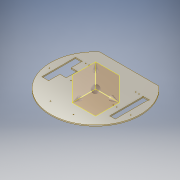
# Autodesk Inventor part: BottomPlate
Saved by Autodesk Inventor 2019 (Build 230136000, 136)
## iProperties
Created: 2020-02-28
Part Number: BottomPlate
Material: Generic
Document SubType Name: Modeling
Designer: james
Mass: 617.778 g
Surface Area: 2655.15 cm^2
Volume: 617.778 cm^3
Density: 1 g/cm^3
Appearance: Titanium
Author: james
Autodesk Inventor part; units mm, degrees
ref_plane "YZ Plane" through (0, 0, 0) normal (1, 0, 0) x (0, 1, 0)
ref_plane "XZ Plane" through (0, 0, 0) normal (0, 1, 0) x (-1, 0, 0)
ref_plane "XY Plane" through (0, 0, 0) normal (0, 0, 1) x (1, 0, 0)
sketch "Sketch1" plane through (0, 0, 0) normal (0, 1, 0) x (-1, 0, 0)
  circle A0 centre (0, 0) radius 203.2
  dimension "d0" = 406.4
  constraints: 1 centre point, 1 coincident
  measures "d0" diameter of A0
extrude "Extrusion1" add sketch "Sketch1" along normal blind 4.7625
sketch "Sketch2" plane through (0, 4.7625, 0) normal (0, 1, 0) x (1, 0, 0)
  line L0 (-165.1, -76.2) -> (-139.7, -76.2)
  line L1 (-139.7, -76.2) -> (-139.7, 76.2)
  line L2 (-139.7, 76.2) -> (-165.1, 76.2)
  line L3 (-165.1, 76.2) -> (-165.1, -76.2)
  line L4 (139.7, 76.2) -> (165.1, 76.2)
  line L5 (165.1, 76.2) -> (165.1, -76.2)
  line L6 (165.1, -76.2) -> (139.7, -76.2)
  line L7 (139.7, -76.2) -> (139.7, 76.2)
  point P0 (0, 0)
  dimension "d3" = 25.4
  dimension "d4" = 25.4
  dimension "d5" = 0
  dimension "d6" = 0
  dimension "d7" = 152.4
  dimension "d8" = 76.2
  dimension "d9" = 139.7
  dimension "d10" = 139.7
  constraints: 16 end point, 4 parallel, 2 horizontal, 2 perpendicular
  measures "d3" distance of L5.end L6.end
  measures "d4" distance of L0.start L0.end
  measures "d5" distance between parallel lines of L6 L0
  measures "d6" distance between parallel lines of L4 L2
  measures "d7" distance of L4.end L5.end
  measures "d8" distance from line of point (0, 0) L6
  measures "d9" distance from line of L1 point (0, 0)
  measures "d10" distance from line of L7 point (0, 0)
extrude "Extrusion2" cut sketch "Sketch2" against normal blind 28.575
sketch "Sketch3" plane through (0, 4.7625, 0) normal (0, 1, 0) x (1, 0, 0)
  line L0 (-139.7, 76.2) -> (-139.7, -76.2) projected
  line L1 (-139.7, -76.2) -> (-165.1, -76.2) projected
  line L2 (-139.7, 76.2) -> (-165.1, 76.2) projected
  point P0 (0, 0)
  point P1 (-120.65, 76.2)
  dimension "d30" = 0
  dimension "d90" = 19.05
  measures "d30" distance from line of point (-120.65, 76.2) L2
  measures "d90" distance from line of L0 point (-120.65, 76.2)
hole "Hole1" at (-120.65, 4.7625, -76.2) direction (0, -1, 0) diameter 3.81 depth 25.4 tip angle 118
sketch "Sketch4" plane through (0, 0, 0) normal (0, -1, 0) x (1, 0, 0)
  line L0 (-136.525, 76.2) -> (-167.64, 76.2)
  line L1 (-167.64, 76.2) -> (-167.64, -76.2)
  line L2 (-167.64, -76.2) -> (-136.525, -76.2)
  line L3 (-136.525, -76.2) -> (-136.525, 76.2)
  line L4 (-139.7, -76.2) -> (-165.1, -76.2) projected
  line L5 (-165.1, 76.2) -> (-139.7, 76.2) projected
  line L6 (-165.1, -76.2) -> (-165.1, 76.2) projected
  line L7 (-139.7, 76.2) -> (-139.7, -76.2) projected
  point P0 (0, 0)
  dimension "d24" = 0
  dimension "d25" = 0
  dimension "d26" = 2.54
  dimension "d27" = 3.175
  constraints: 8 end point, 2 parallel, 1 horizontal, 1 perpendicular
  measures "d24" distance between parallel lines of L2 L4
  measures "d25" distance between parallel lines of L5 L0
  measures "d26" distance between parallel lines of L6 L1
  measures "d27" distance between parallel lines of L7 L3
extrude "Extrusion3" cut sketch "Sketch4" against normal blind 11.1125 contours L3 L2 L7 L0 | L6 L2 L1 L0
sketch "Sketch5" plane through (0, 0, 0) normal (0, -1, 0) x (1, 0, 0)
  circle A0 centre (-120.65, 25.4) radius 1.905 projected
  circle A1 centre (-120.65, -76.2) radius 1.905 projected
  point P0 (0, 0)
  point P1 (-86.36, 25.4)
  point P2 (-105.41, -76.2)
  point P3 (-184.15, 25.4)
  dimension "d33" = 0
  dimension "d34" = 15.24
  dimension "d88" = 101.6
  dimension "d91" = 97.79
  measures "d33" vertical distance of A1.centre point (-105.41, -76.2)
  measures "d34" distance of A1.centre point (-105.41, -76.2)
  measures "d88" vertical distance of point (-184.15, 25.4) A1.centre
  measures "d91" distance of point (-184.15, 25.4) point (-86.36, 25.4)
hole "Hole2" at (-86.36, 0, 25.4) at (-105.41, 0, -76.2) at (-184.15, 0, 25.4) direction (0, 1, 0) diameter 3.81 depth 25.4 tip angle 118
sketch "Sketch6" plane through (0, 0, 0) normal (0, -1, 0) x (1, 0, 0)
  point P0 (0, 0)
  point P1 (52.197, 152.4)
  point P2 (-52.197, 152.4)
  dimension "d48" = 0
  dimension "d49" = 104.394
  dimension "d50" = 52.197
  dimension "d51" = 152.4
  measures "d48" vertical distance of point (-52.197, 152.4) point (52.197, 152.4)
  measures "d49" distance of point (-52.197, 152.4) point (52.197, 152.4)
  measures "d50" horizontal distance of point (0, 0) point (52.197, 152.4)
  measures "d51" vertical distance of point (0, 0) point (-52.197, 152.4)
hole "Hole3" at (52.197, 0, 152.4) at (-52.197, 0, 152.4) direction (0, 1, 0) diameter 3.81 depth 25.4 tip angle 118
sketch "Sketch7" plane through (0, 0, 0) normal (0, -1, 0) x (1, 0, 0)
  circle A0 centre (-86.36, 25.4) radius 1.905 projected
  circle A1 centre (-120.65, 25.4) radius 1.905 projected
  line L0 (139.7, -76.2) -> (139.7, 76.2) projected
  circle A2 centre (-105.41, -76.2) radius 1.905 projected
  point P0 (0, 0)
  point P1 (120.65, 25.4)
  point P2 (105.41, 25.4)
  point P3 (184.15, 25.4)
  point P4 (165.1, -76.2)
  point P5 (139.7, -76.2)
  point P6 (120.65, -76.2)
  point P7 (105.41, -76.2)
  dimension "d59" = 0
  dimension "d60" = 0
  dimension "d61" = 15.24
  dimension "d62" = 63.5
  dimension "d63" = 0
  dimension "d64" = 19.05
  dimension "d65" = 0
  dimension "d66" = 0
  dimension "d67" = 0
  dimension "d68" = 0
  dimension "d69" = 15.24
  dimension "d70" = 19.05
  dimension "d71" = 25.4
  dimension "d72" = 0
  measures "d59" vertical distance of point (120.65, 25.4) point (184.15, 25.4)
  measures "d60" vertical distance of point (105.41, 25.4) point (120.65, 25.4)
  measures "d61" distance of point (105.41, 25.4) point (120.65, 25.4)
  measures "d62" distance of point (184.15, 25.4) point (120.65, 25.4)
  measures "d63" vertical distance of point (105.41, 25.4) A0.centre
  measures "d64" distance from line of point (120.65, 25.4) L0
  measures "d65" vertical distance of point (105.41, -76.2) point (120.65, -76.2)
  measures "d66" vertical distance of point (120.65, -76.2) point (139.7, -76.2)
  measures "d67" vertical distance of point (139.7, -76.2) point (165.1, -76.2)
  measures "d68" vertical distance of point (165.1, -76.2) A2.centre
  measures "d69" distance of point (105.41, -76.2) point (120.65, -76.2)
  measures "d70" distance of point (139.7, -76.2) point (120.65, -76.2)
  measures "d71" distance of point (139.7, -76.2) point (165.1, -76.2)
  measures "d72" horizontal distance of point (120.65, 25.4) point (120.65, -76.2)
hole "Hole4" at (120.65, 0, 25.4) at (105.41, 0, 25.4) at (184.15, 0, 25.4) at (165.1, 0, -76.2) at (139.7, 0, -76.2) at (120.65, 0, -76.2) at (105.41, 0, -76.2) direction (0, 1, 0) diameter 3.81 depth 25.4 tip angle 118
sketch "Sketch8" plane through (0, 4.7625, 0) normal (0, 1, 0) x (1, 0, 0)
  line L0 (-249.9736, 258.2829) -> (238.9858, 258.2829)
  line L1 (238.9858, 258.2829) -> (238.9858, 152.4)
  line L2 (238.9858, 152.4) -> (-249.9736, 152.4)
  line L3 (-249.9736, 152.4) -> (-249.9736, 258.2829)
  point P0 (0, 0)
  dimension "d80" = 152.4
  constraints: 8 end point, 2 parallel, 1 horizontal, 1 perpendicular
  measures "d80" distance from line of point (0, 0) L2
extrude "Extrusion4" cut sketch "Sketch8" against normal blind 100.0125
sketch "Sketch9" plane through (0, 4.7625, 0) normal (0, 1, 0) x (1, 0, 0)
  line L0 (-145.9264, 25.4) -> (-107.95, 25.4)
  line L1 (-107.95, 25.4) -> (-107.95, -25.4)
  line L2 (-107.95, -25.4) -> (-145.9264, -25.4)
  line L3 (-145.9264, -25.4) -> (-145.9264, 25.4)
  line L4 (-136.525, 76.2) -> (-136.525, -76.2) projected
  line L5 (-167.64, 76.2) -> (-136.525, 76.2) projected
  point P0 (0, 0)
  dimension "d83" = 50.8
  dimension "d84" = 28.575
  dimension "d85" = 50.8
  constraints: 8 end point, 2 parallel, 1 horizontal, 1 perpendicular
  measures "d83" distance of L0.end L1.end
  measures "d84" distance between parallel lines of L4 L1
  measures "d85" distance between parallel lines of L5 L0
extrude "Extrusion5" cut sketch "Sketch9" against normal blind 9.525
body "Solid1"
